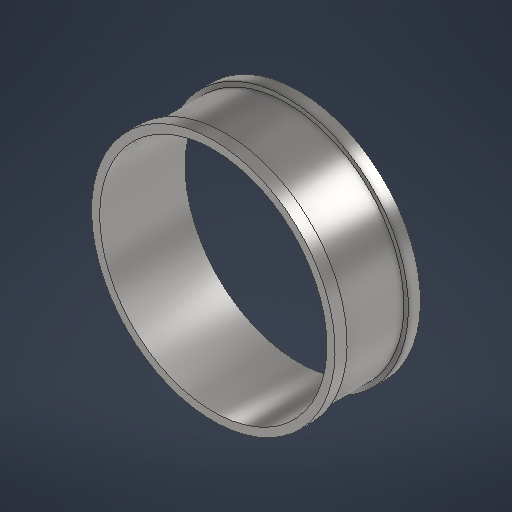
# Autodesk Inventor part: DiscoCorpoTurbina4
Saved by Autodesk Inventor 2026.2 (Build 302298010, 298A)
## iProperties
Created: 2026-04-30
Part Number: DiscoCorpoTurbina4
Material: Steel, Alloy
Document SubType Name: Modeling
Designer: Yan
Density: 7.73 g/cm^3
Appearance: Semi-Polished
Author: Yan
Autodesk Inventor part; units mm, degrees
ref_plane "YZ Plane" through (0, 0, 0) normal (1, 0, 0) x (0, 1, 0)
ref_plane "XZ Plane" through (0, 0, 0) normal (0, 1, 0) x (-1, 0, 0)
ref_plane "XY Plane" through (0, 0, 0) normal (0, 0, 1) x (1, 0, 0)
sketch "Sketch1" plane through (0, 0, 0) normal (1, 0, 0) x (0, 1, 0)
  line L0 (0, 0) -> (0, -284)
  line L1 (0, 0) -> (378, 0)
  line L2 (378, 0) -> (378, -284)
  line L3 (378, -284) -> (0, -284)
  line L4 (378, 0) -> (405, 0)
  line L5 (405, 0) -> (405, -40)
  line L6 (405, -40) -> (390, -40)
  line L7 (390, -40) -> (390, -244)
  line L8 (390, -244) -> (405, -244)
  line L9 (405, -244) -> (405, -284)
  line L10 (378, -284) -> (405, -284)
  dimension "d0" = 756
  dimension "d1" = 780
  dimension "d2" = 810
  dimension "d3" = 40
  dimension "d4" = 40
  dimension "d5" = 284
  constraints: 22 end point, 7 perpendicular, 4 point on line, 1 horizontal, 1 vertical
  measures "d0" diameter of L2 L0
  measures "d1" diameter of L7 L0
  measures "d2" diameter of L5 L0
  measures "d3" distance between parallel lines of L4 L6
  measures "d4" distance between parallel lines of L10 L8
  measures "d5" distance of L0.start L0.end
revolve "Revolution1" add sketch "Sketch1" angle 360 about axis through (0, 0, 0) along (0, 0, -1) contours L4 L5 L6 L7 L8 L9 L10 L2
body "Solid1"
